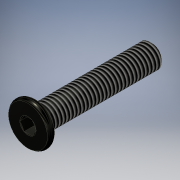
# Autodesk Inventor part: Low Profile Screw M5 [25mm]
Saved by Autodesk Inventor 2019 (Build 230136000, 136)
## iProperties
Created: 2020-11-22
Part Number: Low Profile Screw M5 [25mm]
Material: Steel
Document SubType Name: Modeling
Designer: asus
Density: 7.85 g/cm^3
Appearance: Gunmetal
Author: asus
Autodesk Inventor part; units mm, degrees
ref_plane "YZ Plane" through (0, 0, 0) normal (1, 0, 0) x (0, 1, 0)
ref_plane "XZ Plane" through (0, 0, 0) normal (0, 1, 0) x (-1, 0, 0)
ref_plane "XY Plane" through (0, 0, 0) normal (0, 0, 1) x (1, 0, 0)
sketch "Sketch1" plane through (0, 0, 0) normal (1, 0, 0) x (0, 1, 0)
  line L0 (2.5, 2.81) -> (2.5, 11.31)
  spline S0 degree 2 poles (-3.9658, 2.81) (-4.0258, 2.8689) (-4.0876, 2.9295) knots 0 0 0 0.017848 0.017848 0.017848 weights 1 1.00044 1.00066
  line L1 (-2.5, 11.31) -> (-2.5, 2.81)
  line L2 (1.7321, 14.76) -> (1.7821, 14.81)
  line L3 (-1.7821, 14.81) -> (4.1614, 14.81)
  arc A0 (4.1614, 13.31) -> (4.1614, 14.81) centre (3.5, 14.06) ccw
  line L4 (4.1614, 13.31) -> (2.5, 13.31)
  line L5 (2.5, 13.31) -> (2.5, -11.19)
  line L6 (2.5, -11.19) -> (2, -11.69)
  line L7 (2, -11.69) -> (-2, -11.69)
  line L8 (-2, -11.69) -> (-2.5, -11.19)
  line L9 (-2.5, -11.19) -> (-2.5, 13.31)
  line L10 (-2.5, 13.31) -> (-4.1614, 13.31)
  arc A1 (-4.1614, 14.81) -> (-4.1614, 13.31) centre (-3.5, 14.06) ccw
  line L11 (-4.1614, 14.81) -> (-1.7821, 14.81)
  line L12 (-1.7821, 14.81) -> (-1.7321, 14.76)
  line L13 (-2, -11.69) -> (2, -11.69)
  line L14 (0, -11.69) -> (0, 14.81)
  point P0 (0, 0)
  constraints: 30 end point, 4 point on circle, 2 centre point, 2 point on line, 1 midpoint, 1 vertical, 3 other
revolve "Revolution1" add sketch "Sketch1" angle 360 about axis through (0, 0, -11.69) along (0, 0, 1) contours L5 L6 L7 L14 L3 A0 L4 L0
sketch "Sketch2" plane through (0, 0, 14.81) normal (0, 0, 1) x (1, 0, 0)
  line L0 (1.732, 0) -> (0.866, -1.5)
  line L1 (0.866, -1.5) -> (-0.866, -1.5)
  line L2 (-0.866, -1.5) -> (-1.732, 0)
  line L3 (-1.732, 0) -> (-0.866, 1.5)
  line L4 (-0.866, 1.5) -> (0.866, 1.5)
  line L5 (0.866, 1.5) -> (1.732, 0)
  point P0 (0, 0)
  point P1 (0, 0)
  dimension "d1" = 3.464
  constraints: 12 end point, 1 coincident, 13 other
  measures "d1" distance of L2.end L0.start
extrude "Extrusion1" cut sketch "Sketch2" against normal blind 2.3
sketch "Sketch3" plane through (0, 0, 0) normal (0, 1, 0) x (-1, 0, 0)
  line L0 (0.866, 14.81) -> (-0.866, 14.81) projected
  line L1 (0.866, 14.81) -> (0.866, 12.51) projected
  line L2 (0.866, 12.51) -> (-0.866, 12.51) projected
  line L3 (-0.866, 14.81) -> (-0.866, 12.51) projected
  line L4 (1.732, 14.81) -> (1.732, 12.51) projected
  circle A0 centre (0, 19.6597) radius 5.1497
  line L5 (0, 14.81) -> (0, 14.51)
  line L6 (0, 14.81) -> (0, 24.8094)
  point P0 (0, 0)
  dimension "d5" = 0.3
  constraints: 4 end point, 3 point on circle, 2 vertical, 1 centre point, 1 midpoint, 1 vertical alignment
  measures "d5" distance of L5.start L5.end
revolve "Revolution2" cut sketch "Sketch3" angle 360 about axis through (0, 0, 14.81) along (0, 0, 1) contours L5 A0 L3 L0 | L0 L3 A0 L6
thread "Thread1" size "M5x0.8" class "6g" standard "ANSI Metric M Profile" full length
body "Solid1"
